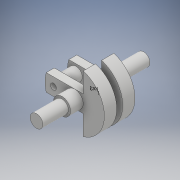
# Autodesk Inventor part: crank
Saved by Autodesk Inventor 2018 (Build 220112000, 112)
## iProperties
Created: 2018-11-06
Part Number: crank
Material: Generic
Document SubType Name: Modeling
Designer: HP
Density: 1 g/cm^3
Appearance: Default
Author: HP
Autodesk Inventor part; units mm, degrees
ref_plane "YZ Plane" through (0, 0, 0) normal (1, 0, 0) x (0, 1, 0)
ref_plane "XZ Plane" through (0, 0, 0) normal (0, 1, 0) x (-1, 0, 0)
sketch "Sketch1" plane through (0, 0, 0) normal (0, 1, 0) x (-1, 0, 0)
  arc A0 (-20.2731, 67) -> (-20.2731, -67) centre (0, 0) ccw
  line L0 (0, 67) -> (0, -67)
  line L1 (0, -67) -> (-20.2731, -67)
  line L2 (-20.2731, 67) -> (-20.2731, -67)
  line L3 (-20.2731, 0) -> (-0.2731, 0)
  circle A1 centre (-0.2731, 0) radius 20
  circle A2 centre (-0.2731, 0) radius 15
  line L4 (-20.2731, 20) -> (69.7269, 20)
  arc A3 (66.8089, -20) -> (66.8089, 20) centre (-0.2731, 0) ccw
  line L5 (-20.2731, -20) -> (66.8089, -20)
  dimension "d0" = 140
  dimension "d1" = 134
  dimension "d2" = 20
  dimension "d3" = 30
  dimension "d4" = 90
  constraints: 12 end point, 4 coincident, 4 perpendicular, 4 point on circle, 3 centre point, 3 point on line, 1 horizontal, 1 horizontal alignment, 1 midpoint, 1 vertical, 2 other
  measures "d0" diameter of A0
  measures "d1" distance of L0.start L0.end
  measures "d2" distance of L3.start L3.end
  measures "d3" diameter of A2
  measures "d4" distance of L4.start L4.end
extrude "Extrusion1" add sketch "Sketch1" against normal blind 29 contours L2 A0 | L4 A1 L2 | L2 A1 L5 | A1 L0 A2 L3 | L3 A2 L0 A1 | A1 L0 A2 | L4 A3 L5 A1 | A2 L0 | A2 L0
sketch "Sketch2" plane through (0, 0, 0) normal (0, 1, 0) x (1, 0, 0)
  line L0 (-66.8089, 20) -> (20.2731, 20) projected
  line L1 (20.2731, -20.1759) -> (20.2731, 20)
  line L2 (20.2731, -20.1759) -> (-74.6075, -20.1759)
  line L3 (-74.6075, -20.1759) -> (-74.6075, 20)
  line L4 (-74.6075, 20) -> (20.2731, 20)
  line L5 (20.2731, 20) -> (20.2731, -20.1759)
  point P0 (0, 0)
  constraints: 10 end point, 2 parallel, 1 horizontal, 1 perpendicular, 1 point on line, 1 vertical
extrude "Extrusion2" cut sketch "Sketch2" against normal blind 10
ref_plane "Work Plane1" through (0, 7, 0) normal (0, 1, 0) x (1, 0, 0)
sketch "Sketch3" plane through (0, -29, 0) normal (0, -1, 0) x (1, 0, 0)
  line L0 (20.2731, -67) -> (20.2731, 67) projected
  line L1 (20.2731, 0) -> (0.2731, 0)
  circle A0 centre (0.2731, 0) radius 20
  point P0 (0, 0)
  dimension "d10" = 20
  constraints: 2 end point, 1 coincident, 1 horizontal, 1 horizontal alignment, 1 midpoint, 2 other
  measures "d10" distance of L1.start L1.end
extrude "Extrusion3" add sketch "Sketch3" along normal blind 30
sketch "Sketch4" plane through (0.2731, -59, 0) normal (0, -1, 0) x (1, 0, 0)
  point P0 (-0.2731, 0)
sketch "Sketch5" plane through (0, -29, 0) normal (0, -1, 0) x (1, 0, 0)
  line L0 (20.2731, -67) -> (20.2731, 67) projected
  line L1 (20.2731, 0) -> (0.2731, 0)
  circle A0 centre (0.2731, 0) radius 15
  point P0 (0, 0)
  dimension "d13" = 20
  dimension "d14" = 30
  constraints: 2 end point, 1 centre point, 1 coincident, 1 horizontal, 1 midpoint
  measures "d13" distance of L1.start L1.end
  measures "d14" diameter of A0
extrude "Extrusion4" add sketch "Sketch5" along normal blind 90
sketch "Sketch6" plane through (0, 0, 0) normal (0, 1, 0) x (1, 0, 0)
  point P0 (0, 0)
sketch "Sketch7" plane through (0, -10, 0) normal (0, 1, 0) x (1, 0, 0)
  line L0 (20.2731, 67) -> (20.2731, -67) projected
  line L1 (20.2731, 0) -> (-49.7269, 0)
  circle A0 centre (-49.7269, 0) radius 15
  point P0 (0, 0)
  dimension "d17" = 70
  dimension "d18" = 30
  constraints: 2 end point, 1 centre point, 1 coincident, 1 horizontal, 1 midpoint
  measures "d17" distance of L1.start L1.end
  measures "d18" diameter of A0
extrude "Extrusion5" add sketch "Sketch7" along normal blind 17
mirror "Mirror1" about plane through (0, 7, 0) normal (0, 1, 0) of "Extrusion1", "Extrusion5", "Extrusion3", "Extrusion4", "Extrusion2"
hole "Hole1" at (-49.7269, 43, 0) direction (0, -1, 0) diameter 14 end through all
sketch "Sketch8" plane through (0, 7, 0) normal (0, 1, 0) x (1, 0, 0)
  arc A0 (0.2731, -20) -> (0.2731, 20) centre (0.2731, 0) ccw projected
  line L0 (20.2731, 0) -> (0.2731, 0)
  circle A1 centre (0.2731, 0) radius 15
  point P0 (0, 0)
  dimension "d30" = 20
  constraints: 2 end point, 1 centre point, 1 coincident, 1 horizontal, 1 point on circle
  measures "d30" distance of L0.start L0.end
body "Solid1"
